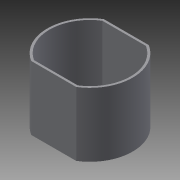
# Autodesk Inventor part: alternate brain box
Saved by Autodesk Inventor 2015 (Build 190159000, 159)
## iProperties
Created: 2014-10-12
Part Number: alternate brain box
Material: Generic
Document SubType Name: Modeling
Designer: ericd_000
Density: 1 g/cm^3
Appearance: Default
Author: ericd_000
Autodesk Inventor part; units mm, degrees
ref_plane "YZ Plane" through (0, 0, 0) normal (1, 0, 0) x (0, 1, 0)
ref_plane "XZ Plane" through (0, 0, 0) normal (0, 1, 0) x (-1, 0, 0)
ref_plane "XY Plane" through (0, 0, 0) normal (0, 0, 1) x (1, 0, 0)
sketch "Sketch1" plane through (0, 0, 0) normal (0, 0, 1) x (1, 0, 0)
  circle A0 centre (0, 0) radius 100
  dimension "d0" = 200
  constraints: 1 centre point, 1 coincident
  measures "d0" diameter of A0
extrude "Extrusion1" add sketch "Sketch1" along normal blind 150
sketch "Sketch3" plane through (0, 0, 150) normal (0, 0, 1) x (1, 0, 0)
  line L0 (0, 0) -> (0, 85) construction
  circle A0 centre (0, 0) radius 100 projected
  arc A1 (52.6783, 85) -> (-52.6783, 85) centre (0, 0) ccw
  line L1 (52.6783, 85) -> (-52.6783, 85)
  dimension "d4" = 85
  constraints: 4 end point, 4 point on circle, 1 centre point, 1 coincident, 1 concentric, 1 midpoint, 1 perpendicular, 1 vertical
  measures "d4" distance of L0.start L0.end
extrude "Extrusion2" cut sketch "Sketch3" against normal up to surface (150 mm away) contours L1 A0 picked at (-13.4735, 87.1556)
mirror "Mirror1" about plane through (0, 0, 0) normal (0, 1, 0) of "Extrusion2"
shell "Shell1" thickness 5 removed faces 1 at (-13.8939, 25.7023, 150)
body "Solid1"
